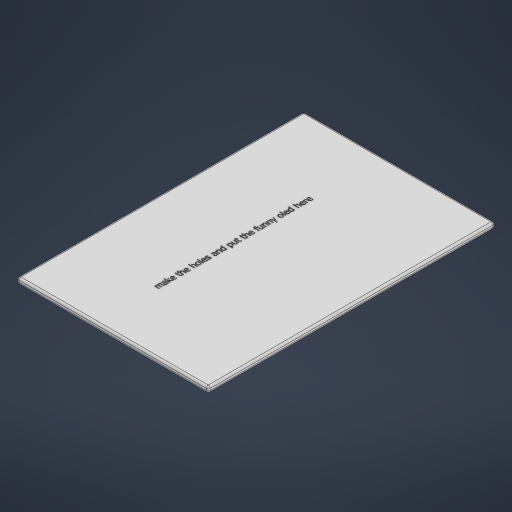
# Autodesk Inventor part: ecu-box-lid
Saved by Autodesk Inventor 2024.2 (Build 282272000, 272)
## iProperties
Created: 2025-06-20
Part Number: ecu-box-lid
Material: Generic
Document SubType Name: Modeling
Designer: Moe
Density: 1 g/cm^3
Appearance: Default
Author: Moe
Autodesk Inventor part; units mm, degrees
(part 1 of 2)
ref_plane "YZ Plane" through (0, 0, 0) normal (1, 0, 0) x (0, 1, 0)
ref_plane "XZ Plane" through (0, 0, 0) normal (0, 1, 0) x (-1, 0, 0)
ref_plane "XY Plane" through (0, 0, 0) normal (0, 0, 1) x (1, 0, 0)
sketch "Sketch1" plane through (0, 0, 0) normal (0, 1, 0) x (-1, 0, 0)
  line L0 (0, 0) -> (100, 0)
  line L1 (100, 0) -> (100, -150)
  line L2 (100, -150) -> (0, -150)
  line L3 (0, -150) -> (0, 0)
  dimension "d0" = 100
  dimension "d1" = 150
  constraints: 8 end point, 2 parallel, 1 horizontal, 1 perpendicular
  measures "d0" distance of L1.end L2.end
  measures "d1" distance of L0.end L1.end
extrude "Extrusion1" add sketch "Sketch1" along normal blind 3
sketch "Sketch2" plane through (0, 0, 0) normal (0, -1, 0) x (1, 0, 0)
  line L0 (0, -150) -> (-100, -150) projected
  line L1 (0, 0) -> (0, -150) projected
  line L2 (-100, 0) -> (0, 0) projected
  line L3 (-100, -150) -> (-100, 0) projected
  line L4 (-5.25, -3.25) -> (-94.75, -3.25)
  line L5 (-96.75, -5.25) -> (-96.75, -144.75)
  line L6 (-94.75, -146.75) -> (-5.25, -146.75)
  line L7 (-3.25, -144.75) -> (-3.25, -5.25)
  arc A0 (-3.25, -5.25) -> (-5.25, -3.25) centre (-5.25, -5.25) ccw
  arc A1 (-94.75, -3.25) -> (-96.75, -5.25) centre (-94.75, -5.25) ccw
  arc A2 (-96.75, -144.75) -> (-94.75, -146.75) centre (-94.75, -144.75) ccw
  arc A3 (-5.25, -146.75) -> (-3.25, -144.75) centre (-5.25, -144.75) ccw
  line L8 (-8.25, -6.25) -> (-91.75, -6.25)
  line L9 (-93.75, -8.25) -> (-93.75, -141.75)
  line L10 (-91.75, -143.75) -> (-8.25, -143.75)
  line L11 (-6.25, -141.75) -> (-6.25, -8.25)
  arc A4 (-6.25, -8.25) -> (-8.25, -6.25) centre (-8.25, -8.25) ccw
  arc A5 (-8.25, -143.75) -> (-6.25, -141.75) centre (-8.25, -141.75) ccw
  arc A6 (-93.75, -141.75) -> (-91.75, -143.75) centre (-91.75, -141.75) ccw
  arc A7 (-91.75, -6.25) -> (-93.75, -8.25) centre (-91.75, -8.25) ccw
  point P0 (-3.25, -3.25)
  point P1 (-96.75, -146.75)
  point P2 (-96.75, -3.25)
  point P3 (-3.25, -146.75)
  point P4 (-50, -143.75)
  dimension "d4" = 3.25
  dimension "d5" = 3.25
  dimension "d6" = 3.25
  dimension "d7" = 3.25
  dimension "d10" = 2
  dimension "d12" = 3
  dimension "d13" = 3
  dimension "d14" = 3
  dimension "d15" = 3
  dimension "d16" = 2
  constraints: 16 end point, 16 point on circle, 16 tangent, 8 centre point, 8 point on line, 6 equal radius, 4 parallel, 2 horizontal, 2 perpendicular, 1 midpoint
  measures "d4" distance between parallel lines of L1 L7
  measures "d5" distance between parallel lines of L3 L5
  measures "d6" distance between parallel lines of L2 L4
  measures "d7" distance between parallel lines of L0 L6
  measures "d10" radius of A0
  measures "d12" distance between parallel lines of L7 L11
  measures "d13" distance between parallel lines of L4 L8
  measures "d14" distance between parallel lines of L5 L9
  measures "d15" distance from line of L6 point (-50, -143.75)
  measures "d16" radius of A4
extrude "Extrusion2" add sketch "Sketch2" along normal blind 3 contours A0 L7 A3 L6 A2 L5 A1 L4
fillet "Fillet1" radius 1 20 edges at (-50, 0, 0) (0, 1.5, 0) (0, 0, -75) (0, 3, -75) (-50, 3, 0) (-3.8358, -3, -3.8358) (-50, -3, -3.25) (-96.1642, -3, -3.8358) (-96.75, -3, -75) (-96.1642, -3, -146.1642) (-50, -3, -146.75) (-3.8358, -3, -146.1642) (-3.25, -3, -75) (0, 1.5, -150) (-50, 3, -150) (-50, 0, -150) (-100, 3, -75) (-100, 1.5, -150) (-100, 0, -75) (-100, 1.5, 0)
sketch "Sketch3" plane through (0, 3, 0) normal (0, 1, 0) x (1, 0, 0)
  line L0 (-60.8151, 31.4553) -> (-60.8151, 114.1441) construction
  line L1 (-60.8151, 114.1441) -> (-56.7693, 114.1441) construction
  line L2 (-56.7693, 114.1441) -> (-56.7693, 31.4553) construction
  line L3 (-56.7693, 31.4553) -> (-60.8151, 31.4553) construction
  line L4 (-57.6115, 34.328) -> (-58.9355, 34.328)
  spline S0 degree 2 poles (-58.9355, 34.328) (-59.0935, 34.328) (-59.3628, 34.3033) (-59.4369, 34.2637) knots 0 0 0 1 2 2 2
  spline S1 degree 2 poles (-59.4369, 34.2637) (-59.5184, 34.2242) (-59.5974, 34.0735) (-59.5974, 33.9426) knots 0 0 0 1 2 2 2
  spline S2 degree 2 poles (-59.5974, 33.9426) (-59.5974, 33.8241) (-59.4517, 33.5524) (-59.3134, 33.4091) knots 0 0 0 1 2 2 2
  spline S3 degree 2 poles (-59.3134, 33.4091) (-59.2788, 33.4116) (-59.1825, 33.4165) (-59.1182, 33.4165) knots 0 0 0 1 2 2 2
  line L5 (-59.1182, 33.4165) -> (-57.6115, 33.4165)
  line L6 (-57.6115, 33.4165) -> (-57.6115, 33.0312)
  line L7 (-57.6115, 33.0312) -> (-58.9355, 33.0312)
  spline S4 degree 2 poles (-58.9355, 33.0312) (-59.0935, 33.0312) (-59.3628, 33.0065) (-59.4369, 32.967) knots 0 0 0 1 2 2 2
  spline S5 degree 2 poles (-59.4369, 32.967) (-59.5184, 32.9275) (-59.5974, 32.7768) (-59.5974, 32.6459) knots 0 0 0 1 2 2 2
  spline S6 degree 2 poles (-59.5974, 32.6459) (-59.5974, 32.5224) (-59.4418, 32.2482) (-59.3208, 32.1198) knots 0 0 0 1 2 2 2
  line L8 (-59.3208, 32.1198) -> (-57.6115, 32.1198)
  line L9 (-57.6115, 32.1198) -> (-57.6115, 31.7344)
  line L10 (-57.6115, 31.7344) -> (-59.8988, 31.7344)
  line L11 (-59.8988, 31.7344) -> (-59.8988, 32.1198)
  line L12 (-59.8988, 32.1198) -> (-59.6468, 32.1198)
  spline S7 degree 2 poles (-59.6468, 32.1198) (-59.7975, 32.2704) (-59.963, 32.5668) (-59.963, 32.7447) knots 0 0 0 1 2 2 2
  spline S8 degree 2 poles (-59.963, 32.7447) (-59.963, 32.9472) (-59.7777, 33.2609) (-59.5678, 33.3424) knots 0 0 0 1 2 2 2
  spline S9 degree 2 poles (-59.5678, 33.3424) (-59.7629, 33.5178) (-59.963, 33.8488) (-59.963, 34.0414) knots 0 0 0 1 2 2 2
  spline S10 degree 2 poles (-59.963, 34.0414) (-59.963, 34.1896) (-59.8716, 34.4317) (-59.7679, 34.5206) knots 0 0 0 1 2 2 2
  spline S11 degree 2 poles (-59.7679, 34.5206) (-59.6641, 34.612) (-59.3529, 34.7133) (-59.1182, 34.7133) knots 0 0 0 1 2 2 2
  line L13 (-59.1182, 34.7133) -> (-57.6115, 34.7133)
  line L14 (-57.6115, 34.7133) -> (-57.6115, 34.328)
  spline S12 degree 2 poles (-57.8536, 36.5287) (-57.819, 36.4818) (-57.6955, 36.3237) (-57.6585, 36.2496) knots 0 0 0 1 2 2 2
  spline S13 degree 2 poles (-57.6585, 36.2496) (-57.6041, 36.1484) (-57.5473, 35.9582) (-57.5473, 35.7853) knots 0 0 0 1 2 2 2
  spline S14 degree 2 poles (-57.5473, 35.7853) (-57.5473, 35.6445) (-57.6535, 35.3901) (-57.7498, 35.2937) knots 0 0 0 1 2 2 2
  spline S15 degree 2 poles (-57.7498, 35.2937) (-57.8437, 35.2023) (-58.1204, 35.0912) (-58.2735, 35.0912) knots 0 0 0 1 2 2 2
  spline S16 degree 2 poles (-58.2735, 35.0912) (-58.5106, 35.0912) (-58.8465, 35.2913) (-58.9429, 35.5086) knots 0 0 0 1 2 2 2
  spline S17 degree 2 poles (-58.9429, 35.5086) (-59.0318, 35.7013) (-59.0985, 36.2249) (-59.1158, 36.5287) knots 0 0 0 1 2 2 2
  line L15 (-59.1158, 36.5287) -> (-59.1899, 36.5287)
  spline S18 degree 2 poles (-59.1899, 36.5287) (-59.3233, 36.5287) (-59.4887, 36.4472) (-59.5357, 36.3731) knots 0 0 0 1 2 2 2
  spline S19 degree 2 poles (-59.5357, 36.3731) (-59.5826, 36.299) (-59.6122, 36.0866) (-59.6122, 35.973) knots 0 0 0 1 2 2 2
  spline S20 degree 2 poles (-59.6122, 35.973) (-59.6122, 35.8396) (-59.5332, 35.479) (-59.4566, 35.2987) knots 0 0 0 1 2 2 2
  line L16 (-59.4566, 35.2987) -> (-59.4566, 35.2764)
  line L17 (-59.4566, 35.2764) -> (-59.8494, 35.2764)
  spline S21 degree 2 poles (-59.8494, 35.2764) (-59.879, 35.3827) (-59.9531, 35.7803) (-59.9531, 35.9755) knots 0 0 0 1 2 2 2
  spline S22 degree 2 poles (-59.9531, 35.9755) (-59.9531, 36.2126) (-59.879, 36.5361) (-59.7827, 36.6646) knots 0 0 0 1 2 2 2
  spline S23 degree 2 poles (-59.7827, 36.6646) (-59.6888, 36.7906) (-59.3899, 36.9141) (-59.175, 36.9141) knots 0 0 0 1 2 2 2
  line L18 (-59.175, 36.9141) -> (-57.6115, 36.9141)
  line L19 (-57.6115, 36.9141) -> (-57.6115, 36.5287)
  line L20 (-57.6115, 36.5287) -> (-57.8536, 36.5287)
  line L21 (-58.1747, 36.5287) -> (-58.8095, 36.5287)
  spline S24 degree 2 poles (-58.8095, 36.5287) (-58.7971, 36.3904) (-58.7551, 35.973) (-58.7156, 35.8421) knots 0 0 0 1 2 2 2
  spline S25 degree 2 poles (-58.7156, 35.8421) (-58.6687, 35.6889) (-58.4736, 35.4889) (-58.3007, 35.4889) knots 0 0 0 1 2 2 2
  spline S26 degree 2 poles (-58.3007, 35.4889) (-58.1031, 35.4889) (-57.903, 35.7112) (-57.903, 35.9236) knots 0 0 0 1 2 2 2
  spline S27 degree 2 poles (-57.903, 35.9236) (-57.903, 36.1039) (-58.0586, 36.4003) (-58.1747, 36.5287) knots 0 0 0 1 2 2 2
  line L22 (-57.6115, 39.3495) -> (-57.6115, 38.8431)
  line L23 (-57.6115, 38.8431) -> (-58.7156, 37.9935)
  line L24 (-58.7156, 37.9935) -> (-58.5674, 37.8403)
  line L25 (-58.5674, 37.8403) -> (-57.6115, 37.8403)
  line L26 (-57.6115, 37.8403) -> (-57.6115, 37.455)
  line L27 (-57.6115, 37.455) -> (-60.7954, 37.455)
  line L28 (-60.7954, 37.455) -> (-60.7954, 37.8403)
  line L29 (-60.7954, 37.8403) -> (-58.933, 37.8403)
  line L30 (-58.933, 37.8403) -> (-59.8988, 38.7443)
  line L31 (-59.8988, 38.7443) -> (-59.8988, 39.2235)
  line L32 (-59.8988, 39.2235) -> (-58.9429, 38.2849)
  line L33 (-58.9429, 38.2849) -> (-57.6115, 39.3495)
  spline S28 degree 2 poles (-57.5597, 40.5351) (-57.5597, 39.9868) (-58.1747, 39.3841) (-58.7428, 39.3841) knots 0 0 0 1 2 2 2
  spline S29 degree 2 poles (-58.7428, 39.3841) (-59.301, 39.3841) (-59.963, 39.9695) (-59.963, 40.4412) knots 0 0 0 1 2 2 2
  spline S30 degree 2 poles (-59.963, 40.4412) (-59.963, 40.6537) (-59.8395, 40.9822) (-59.7086, 41.1032) knots 0 0 0 1 2 2 2
  spline S31 degree 2 poles (-59.7086, 41.1032) (-59.5777, 41.2267) (-59.1997, 41.3576) (-58.9256, 41.3576) knots 0 0 0 1 2 2 2
  line L34 (-58.9256, 41.3576) -> (-58.7156, 41.3576)
  line L35 (-58.7156, 41.3576) -> (-58.7156, 39.7743)
  spline S32 degree 2 poles (-58.7156, 39.7743) (-58.318, 39.7743) (-57.8956, 40.1745) (-57.8956, 40.5302) knots 0 0 0 1 2 2 2
  spline S33 degree 2 poles (-57.8956, 40.5302) (-57.8956, 40.6561) (-57.9524, 40.9007) (-57.9969, 40.9995) knots 0 0 0 1 2 2 2
  spline S34 degree 2 poles (-57.9969, 40.9995) (-58.0463, 41.1032) (-58.1327, 41.2465) (-58.1722, 41.2934) knots 0 0 0 1 2 2 2
  line L36 (-58.1722, 41.2934) -> (-58.1722, 41.3156)
  line L37 (-58.1722, 41.3156) -> (-57.7523, 41.3156)
  spline S35 degree 2 poles (-57.7523, 41.3156) (-57.7251, 41.2489) (-57.6461, 41.0464) (-57.6239, 40.9674) knots 0 0 0 1 2 2 2
  spline S36 degree 2 poles (-57.6239, 40.9674) (-57.5918, 40.8562) (-57.5597, 40.6734) (-57.5597, 40.5351) knots 0 0 0 1 2 2 2
  spline S37 degree 2 poles (-59.0096, 40.9822) (-59.1652, 40.9772) (-59.3924, 40.913) (-59.469, 40.8513) knots 0 0 0 1 2 2 2
  spline S38 degree 2 poles (-59.469, 40.8513) (-59.5554, 40.7846) (-59.6468, 40.5746) (-59.6468, 40.419) knots 0 0 0 1 2 2 2
  spline S39 degree 2 poles (-59.6468, 40.419) (-59.6468, 40.2659) (-59.5554, 40.051) (-59.4665, 39.9621) knots 0 0 0 1 2 2 2
  spline S40 degree 2 poles (-59.4665, 39.9621) (-59.3751, 39.8756) (-59.1553, 39.7867) (-59.0096, 39.7743) knots 0 0 0 1 2 2 2
  line L38 (-59.0096, 39.7743) -> (-59.0096, 40.9822)
  spline S41 degree 2 poles (-57.5671, 43.7486) (-57.5671, 43.4349) (-57.9252, 43.0817) (-58.313, 43.0817) knots 0 0 0 1 2 2 2
  line L39 (-58.313, 43.0817) -> (-59.5801, 43.0817)
  line L40 (-59.5801, 43.0817) -> (-59.5801, 42.8223)
  line L41 (-59.5801, 42.8223) -> (-59.8988, 42.8223)
  line L42 (-59.8988, 42.8223) -> (-59.8988, 43.0817)
  line L43 (-59.8988, 43.0817) -> (-60.5558, 43.0817)
  line L44 (-60.5558, 43.0817) -> (-60.5558, 43.467)
  line L45 (-60.5558, 43.467) -> (-59.8988, 43.467)
  line L46 (-59.8988, 43.467) -> (-59.8988, 44.1759)
  line L47 (-59.8988, 44.1759) -> (-59.5801, 44.1759)
  line L48 (-59.5801, 44.1759) -> (-59.5801, 43.467)
  line L49 (-59.5801, 43.467) -> (-58.4909, 43.467)
  spline S42 degree 2 poles (-58.4909, 43.467) (-58.318, 43.467) (-58.1278, 43.4794) (-58.0463, 43.5214) knots 0 0 0 1 2 2 2
  spline S43 degree 2 poles (-58.0463, 43.5214) (-57.9746, 43.5559) (-57.903, 43.7115) (-57.903, 43.8449) knots 0 0 0 1 2 2 2
  spline S44 degree 2 poles (-57.903, 43.8449) (-57.903, 43.9388) (-57.9598, 44.1142) (-57.9771, 44.1537) knots 0 0 0 1 2 2 2
  line L50 (-57.9771, 44.1537) -> (-57.9771, 44.1759)
  line L51 (-57.9771, 44.1759) -> (-57.6313, 44.1759)
  spline S45 degree 2 poles (-57.6313, 44.1759) (-57.6016, 44.0672) (-57.5671, 43.8449) (-57.5671, 43.7486) knots 0 0 0 1 2 2 2
  line L52 (-57.6115, 46.2557) -> (-57.6115, 45.8703)
  line L53 (-57.6115, 45.8703) -> (-58.9157, 45.8703)
  spline S46 degree 2 poles (-58.9157, 45.8703) (-59.0738, 45.8703) (-59.3455, 45.8407) (-59.427, 45.7962) knots 0 0 0 1 2 2 2
  spline S47 degree 2 poles (-59.427, 45.7962) (-59.5134, 45.7493) (-59.5974, 45.5813) (-59.5974, 45.4381) knots 0 0 0 1 2 2 2
  spline S48 degree 2 poles (-59.5974, 45.4381) (-59.5974, 45.2948) (-59.4443, 44.991) (-59.3208, 44.8453) knots 0 0 0 1 2 2 2
  line L54 (-59.3208, 44.8453) -> (-57.6115, 44.8453)
  line L55 (-57.6115, 44.8453) -> (-57.6115, 44.46)
  line L56 (-57.6115, 44.46) -> (-60.7954, 44.46)
  line L57 (-60.7954, 44.46) -> (-60.7954, 44.8453)
  line L58 (-60.7954, 44.8453) -> (-59.6444, 44.8453)
  spline S49 degree 2 poles (-59.6444, 44.8453) (-59.8, 45.0182) (-59.963, 45.3516) (-59.963, 45.5394) knots 0 0 0 1 2 2 2
  spline S50 degree 2 poles (-59.963, 45.5394) (-59.963, 45.8753) (-59.5184, 46.2557) (-59.096, 46.2557) knots 0 0 0 1 2 2 2
  line L59 (-59.096, 46.2557) -> (-57.6115, 46.2557)
  spline S51 degree 2 poles (-57.5597, 47.7895) (-57.5597, 47.2412) (-58.1747, 46.6385) (-58.7428, 46.6385) knots 0 0 0 1 2 2 2
  spline S52 degree 2 poles (-58.7428, 46.6385) (-59.301, 46.6385) (-59.963, 47.2239) (-59.963, 47.6957) knots 0 0 0 1 2 2 2
  spline S53 degree 2 poles (-59.963, 47.6957) (-59.963, 47.9081) (-59.8395, 48.2366) (-59.7086, 48.3576) knots 0 0 0 1 2 2 2
  spline S54 degree 2 poles (-59.7086, 48.3576) (-59.5777, 48.4811) (-59.1997, 48.6121) (-58.9256, 48.6121) knots 0 0 0 1 2 2 2
  line L60 (-58.9256, 48.6121) -> (-58.7156, 48.6121)
  line L61 (-58.7156, 48.6121) -> (-58.7156, 47.0288)
  spline S55 degree 2 poles (-58.7156, 47.0288) (-58.318, 47.0288) (-57.8956, 47.4289) (-57.8956, 47.7846) knots 0 0 0 1 2 2 2
  spline S56 degree 2 poles (-57.8956, 47.7846) (-57.8956, 47.9106) (-57.9524, 48.1551) (-57.9969, 48.2539) knots 0 0 0 1 2 2 2
  spline S57 degree 2 poles (-57.9969, 48.2539) (-58.0463, 48.3576) (-58.1327, 48.5009) (-58.1722, 48.5478) knots 0 0 0 1 2 2 2
  line L62 (-58.1722, 48.5478) -> (-58.1722, 48.5701)
  line L63 (-58.1722, 48.5701) -> (-57.7523, 48.5701)
  spline S58 degree 2 poles (-57.7523, 48.5701) (-57.7251, 48.5034) (-57.6461, 48.3008) (-57.6239, 48.2218) knots 0 0 0 1 2 2 2
  spline S59 degree 2 poles (-57.6239, 48.2218) (-57.5918, 48.1106) (-57.5597, 47.9279) (-57.5597, 47.7895) knots 0 0 0 1 2 2 2
  spline S60 degree 2 poles (-59.0096, 48.2366) (-59.1652, 48.2317) (-59.3924, 48.1675) (-59.469, 48.1057) knots 0 0 0 1 2 2 2
  spline S61 degree 2 poles (-59.469, 48.1057) (-59.5554, 48.039) (-59.6468, 47.8291) (-59.6468, 47.6735) knots 0 0 0 1 2 2 2
  spline S62 degree 2 poles (-59.6468, 47.6735) (-59.6468, 47.5203) (-59.5554, 47.3054) (-59.4665, 47.2165) knots 0 0 0 1 2 2 2
  spline S63 degree 2 poles (-59.4665, 47.2165) (-59.3751, 47.13) (-59.1553, 47.0411) (-59.0096, 47.0288) knots 0 0 0 1 2 2 2
  line L64 (-59.0096, 47.0288) -> (-59.0096, 48.2366)
  line L65 (-57.6115, 52.1071) -> (-57.6115, 51.7218)
  line L66 (-57.6115, 51.7218) -> (-58.9157, 51.7218)
  spline S64 degree 2 poles (-58.9157, 51.7218) (-59.0738, 51.7218) (-59.3455, 51.6922) (-59.427, 51.6477) knots 0 0 0 1 2 2 2
  spline S65 degree 2 poles (-59.427, 51.6477) (-59.5134, 51.6008) (-59.5974, 51.4328) (-59.5974, 51.2896) knots 0 0 0 1 2 2 2
  spline S66 degree 2 poles (-59.5974, 51.2896) (-59.5974, 51.1463) (-59.4443, 50.8425) (-59.3208, 50.6968) knots 0 0 0 1 2 2 2
  line L67 (-59.3208, 50.6968) -> (-57.6115, 50.6968)
  line L68 (-57.6115, 50.6968) -> (-57.6115, 50.3114)
  line L69 (-57.6115, 50.3114) -> (-60.7954, 50.3114)
  line L70 (-60.7954, 50.3114) -> (-60.7954, 50.6968)
  line L71 (-60.7954, 50.6968) -> (-59.6444, 50.6968)
  spline S67 degree 2 poles (-59.6444, 50.6968) (-59.8, 50.8697) (-59.963, 51.2031) (-59.963, 51.3908) knots 0 0 0 1 2 2 2
  spline S68 degree 2 poles (-59.963, 51.3908) (-59.963, 51.7267) (-59.5184, 52.1071) (-59.096, 52.1071) knots 0 0 0 1 2 2 2
  line L72 (-59.096, 52.1071) -> (-57.6115, 52.1071)
  spline S69 degree 2 poles (-58.7551, 54.5277) (-58.1772, 54.5277) (-57.5473, 53.972) (-57.5473, 53.5076) knots 0 0 0 1 2 2 2
  spline S70 degree 2 poles (-57.5473, 53.5076) (-57.5473, 53.0309) (-58.1969, 52.485) (-58.7551, 52.485) knots 0 0 0 1 2 2 2
  spline S71 degree 2 poles (-58.7551, 52.485) (-59.3282, 52.485) (-59.963, 53.0482) (-59.963, 53.5076) knots 0 0 0 1 2 2 2
  spline S72 degree 2 poles (-59.963, 53.5076) (-59.963, 53.972) (-59.3307, 54.5277) (-58.7551, 54.5277) knots 0 0 0 1 2 2 2
  spline S73 degree 2 poles (-58.7551, 54.1301) (-59.1997, 54.1301) (-59.632, 53.8065) (-59.632, 53.5076) knots 0 0 0 1 2 2 2
  spline S74 degree 2 poles (-59.632, 53.5076) (-59.632, 53.2088) (-59.1997, 52.8827) (-58.7551, 52.8827) knots 0 0 0 1 2 2 2
  spline S75 degree 2 poles (-58.7551, 52.8827) (-58.3229, 52.8827) (-57.8783, 53.2088) (-57.8783, 53.5076) knots 0 0 0 1 2 2 2
  spline S76 degree 2 poles (-57.8783, 53.5076) (-57.8783, 53.804) (-58.3155, 54.1301) (-58.7551, 54.1301) knots 0 0 0 1 2 2 2
  line L73 (-57.6115, 55.3157) -> (-57.6115, 54.9304)
  line L74 (-57.6115, 54.9304) -> (-60.7954, 54.9304)
  line L75 (-60.7954, 54.9304) -> (-60.7954, 55.3157)
  line L76 (-60.7954, 55.3157) -> (-57.6115, 55.3157)
  spline S77 degree 2 poles (-57.5597, 56.8743) (-57.5597, 56.3259) (-58.1747, 55.7232) (-58.7428, 55.7232) knots 0 0 0 1 2 2 2
  spline S78 degree 2 poles (-58.7428, 55.7232) (-59.301, 55.7232) (-59.963, 56.3086) (-59.963, 56.7804) knots 0 0 0 1 2 2 2
  spline S79 degree 2 poles (-59.963, 56.7804) (-59.963, 56.9928) (-59.8395, 57.3213) (-59.7086, 57.4424) knots 0 0 0 1 2 2 2
  spline S80 degree 2 poles (-59.7086, 57.4424) (-59.5777, 57.5659) (-59.1997, 57.6968) (-58.9256, 57.6968) knots 0 0 0 1 2 2 2
  line L77 (-58.9256, 57.6968) -> (-58.7156, 57.6968)
  line L78 (-58.7156, 57.6968) -> (-58.7156, 56.1135)
  spline S81 degree 2 poles (-58.7156, 56.1135) (-58.318, 56.1135) (-57.8956, 56.5136) (-57.8956, 56.8693) knots 0 0 0 1 2 2 2
  spline S82 degree 2 poles (-57.8956, 56.8693) (-57.8956, 56.9953) (-57.9524, 57.2398) (-57.9969, 57.3386) knots 0 0 0 1 2 2 2
  spline S83 degree 2 poles (-57.9969, 57.3386) (-58.0463, 57.4424) (-58.1327, 57.5856) (-58.1722, 57.6326) knots 0 0 0 1 2 2 2
  line L79 (-58.1722, 57.6326) -> (-58.1722, 57.6548)
  line L80 (-58.1722, 57.6548) -> (-57.7523, 57.6548)
  spline S84 degree 2 poles (-57.7523, 57.6548) (-57.7251, 57.5881) (-57.6461, 57.3856) (-57.6239, 57.3065) knots 0 0 0 1 2 2 2
  spline S85 degree 2 poles (-57.6239, 57.3065) (-57.5918, 57.1954) (-57.5597, 57.0126) (-57.5597, 56.8743) knots 0 0 0 1 2 2 2
  spline S86 degree 2 poles (-59.0096, 57.3213) (-59.1652, 57.3164) (-59.3924, 57.2522) (-59.469, 57.1904) knots 0 0 0 1 2 2 2
  spline S87 degree 2 poles (-59.469, 57.1904) (-59.5554, 57.1237) (-59.6468, 56.9138) (-59.6468, 56.7582) knots 0 0 0 1 2 2 2
  spline S88 degree 2 poles (-59.6468, 56.7582) (-59.6468, 56.605) (-59.5554, 56.3901) (-59.4665, 56.3012) knots 0 0 0 1 2 2 2
  spline S89 degree 2 poles (-59.4665, 56.3012) (-59.3751, 56.2148) (-59.1553, 56.1258) (-59.0096, 56.1135) knots 0 0 0 1 2 2 2
  line L81 (-59.0096, 56.1135) -> (-59.0096, 57.3213)
  spline S90 degree 2 poles (-57.5572, 58.7045) (-57.5572, 58.4748) (-57.6807, 58.0772) (-57.7498, 57.9463) knots 0 0 0 1 2 2 2
  line L82 (-57.7498, 57.9463) -> (-58.1821, 57.9463)
  line L83 (-58.1821, 57.9463) -> (-58.1821, 57.966)
  spline S91 degree 2 poles (-58.1821, 57.966) (-58.1426, 58.0154) (-58.0487, 58.1488) (-57.9969, 58.2599) knots 0 0 0 1 2 2 2
  spline S92 degree 2 poles (-57.9969, 58.2599) (-57.9499, 58.3563) (-57.8808, 58.5934) (-57.8808, 58.7194) knots 0 0 0 1 2 2 2
  spline S93 degree 2 poles (-57.8808, 58.7194) (-57.8808, 58.8108) (-57.9228, 59.0207) (-57.9573, 59.0701) knots 0 0 0 1 2 2 2
  spline S94 degree 2 poles (-57.9573, 59.0701) (-58.0043, 59.1417) (-58.1105, 59.206) (-58.2192, 59.206) knots 0 0 0 1 2 2 2
  spline S95 degree 2 poles (-58.2192, 59.206) (-58.355, 59.206) (-58.4958, 59.0578) (-58.5427, 58.8676) knots 0 0 0 1 2 2 2
  spline S96 degree 2 poles (-58.5427, 58.8676) (-58.56, 58.7935) (-58.6094, 58.5563) (-58.6366, 58.4551) knots 0 0 0 1 2 2 2
  spline S97 degree 2 poles (-58.6366, 58.4551) (-58.7132, 58.1933) (-59.0293, 57.9561) (-59.2541, 57.9561) knots 0 0 0 1 2 2 2
  spline S98 degree 2 poles (-59.2541, 57.9561) (-59.5653, 57.9561) (-59.9531, 58.423) (-59.9531, 58.8083) knots 0 0 0 1 2 2 2
  spline S99 degree 2 poles (-59.9531, 58.8083) (-59.9531, 58.9985) (-59.8592, 59.3838) (-59.7876, 59.5147) knots 0 0 0 1 2 2 2
  line L84 (-59.7876, 59.5147) -> (-59.3751, 59.5147)
  line L85 (-59.3751, 59.5147) -> (-59.3751, 59.495)
  spline S100 degree 2 poles (-59.3751, 59.495) (-59.4937, 59.3467) (-59.6295, 58.9861) (-59.6295, 58.8009) knots 0 0 0 1 2 2 2
  spline S101 degree 2 poles (-59.6295, 58.8009) (-59.6295, 58.6107) (-59.469, 58.3489) (-59.3084, 58.3489) knots 0 0 0 1 2 2 2
  spline S102 degree 2 poles (-59.3084, 58.3489) (-59.1627, 58.3489) (-59.0219, 58.5045) (-58.9774, 58.6774) knots 0 0 0 1 2 2 2
  spline S103 degree 2 poles (-58.9774, 58.6774) (-58.9552, 58.7614) (-58.9108, 58.9738) (-58.8836, 59.0899) knots 0 0 0 1 2 2 2
  spline S104 degree 2 poles (-58.8836, 59.0899) (-58.8194, 59.3418) (-58.5254, 59.5987) (-58.271, 59.5987) knots 0 0 0 1 2 2 2
  spline S105 degree 2 poles (-58.271, 59.5987) (-58.1228, 59.5987) (-57.861, 59.4826) (-57.7647, 59.369) knots 0 0 0 1 2 2 2
  spline S106 degree 2 poles (-57.7647, 59.369) (-57.6634, 59.2479) (-57.5572, 58.9392) (-57.5572, 58.7045) knots 0 0 0 1 2 2 2
  spline S107 degree 2 poles (-57.8536, 62.5405) (-57.819, 62.4936) (-57.6955, 62.3355) (-57.6585, 62.2614) knots 0 0 0 1 2 2 2
  spline S108 degree 2 poles (-57.6585, 62.2614) (-57.6041, 62.1601) (-57.5473, 61.9699) (-57.5473, 61.797) knots 0 0 0 1 2 2 2
  spline S109 degree 2 poles (-57.5473, 61.797) (-57.5473, 61.6562) (-57.6535, 61.4018) (-57.7498, 61.3055) knots 0 0 0 1 2 2 2
  spline S110 degree 2 poles (-57.7498, 61.3055) (-57.8437, 61.2141) (-58.1204, 61.1029) (-58.2735, 61.1029) knots 0 0 0 1 2 2 2
  spline S111 degree 2 poles (-58.2735, 61.1029) (-58.5106, 61.1029) (-58.8465, 61.303) (-58.9429, 61.5204) knots 0 0 0 1 2 2 2
  spline S112 degree 2 poles (-58.9429, 61.5204) (-59.0318, 61.713) (-59.0985, 62.2367) (-59.1158, 62.5405) knots 0 0 0 1 2 2 2
  line L86 (-59.1158, 62.5405) -> (-59.1899, 62.5405)
  spline S113 degree 2 poles (-59.1899, 62.5405) (-59.3233, 62.5405) (-59.4887, 62.459) (-59.5357, 62.3849) knots 0 0 0 1 2 2 2
  spline S114 degree 2 poles (-59.5357, 62.3849) (-59.5826, 62.3108) (-59.6122, 62.0983) (-59.6122, 61.9847) knots 0 0 0 1 2 2 2
  spline S115 degree 2 poles (-59.6122, 61.9847) (-59.6122, 61.8513) (-59.5332, 61.4907) (-59.4566, 61.3104) knots 0 0 0 1 2 2 2
  line L87 (-59.4566, 61.3104) -> (-59.4566, 61.2882)
  line L88 (-59.4566, 61.2882) -> (-59.8494, 61.2882)
  spline S116 degree 2 poles (-59.8494, 61.2882) (-59.879, 61.3944) (-59.9531, 61.7921) (-59.9531, 61.9872) knots 0 0 0 1 2 2 2
  spline S117 degree 2 poles (-59.9531, 61.9872) (-59.9531, 62.2243) (-59.879, 62.5479) (-59.7827, 62.6763) knots 0 0 0 1 2 2 2
  spline S118 degree 2 poles (-59.7827, 62.6763) (-59.6888, 62.8023) (-59.3899, 62.9258) (-59.175, 62.9258) knots 0 0 0 1 2 2 2
  line L89 (-59.175, 62.9258) -> (-57.6115, 62.9258)
  line L90 (-57.6115, 62.9258) -> (-57.6115, 62.5405)
  line L91 (-57.6115, 62.5405) -> (-57.8536, 62.5405)
  line L92 (-58.1747, 62.5405) -> (-58.8095, 62.5405)
  spline S119 degree 2 poles (-58.8095, 62.5405) (-58.7971, 62.4022) (-58.7551, 61.9847) (-58.7156, 61.8538) knots 0 0 0 1 2 2 2
  spline S120 degree 2 poles (-58.7156, 61.8538) (-58.6687, 61.7007) (-58.4736, 61.5006) (-58.3007, 61.5006) knots 0 0 0 1 2 2 2
  spline S121 degree 2 poles (-58.3007, 61.5006) (-58.1031, 61.5006) (-57.903, 61.7229) (-57.903, 61.9353) knots 0 0 0 1 2 2 2
  spline S122 degree 2 poles (-57.903, 61.9353) (-57.903, 62.1156) (-58.0586, 62.412) (-58.1747, 62.5405) knots 0 0 0 1 2 2 2
  line L93 (-57.6115, 65.2624) -> (-57.6115, 64.8771)
  line L94 (-57.6115, 64.8771) -> (-58.9157, 64.8771)
  spline S123 degree 2 poles (-58.9157, 64.8771) (-59.0738, 64.8771) (-59.3455, 64.8475) (-59.427, 64.803) knots 0 0 0 1 2 2 2
  spline S124 degree 2 poles (-59.427, 64.803) (-59.5134, 64.7561) (-59.5974, 64.5881) (-59.5974, 64.4449) knots 0 0 0 1 2 2 2
  spline S125 degree 2 poles (-59.5974, 64.4449) (-59.5974, 64.3016) (-59.4443, 63.9978) (-59.3208, 63.8521) knots 0 0 0 1 2 2 2
  line L95 (-59.3208, 63.8521) -> (-57.6115, 63.8521)
  line L96 (-57.6115, 63.8521) -> (-57.6115, 63.4667)
  line L97 (-57.6115, 63.4667) -> (-59.8988, 63.4667)
  line L98 (-59.8988, 63.4667) -> (-59.8988, 63.8521)
  line L99 (-59.8988, 63.8521) -> (-59.6444, 63.8521)
  spline S126 degree 2 poles (-59.6444, 63.8521) (-59.8, 64.025) (-59.963, 64.3584) (-59.963, 64.5461) knots 0 0 0 1 2 2 2
  spline S127 degree 2 poles (-59.963, 64.5461) (-59.963, 64.8821) (-59.5184, 65.2624) (-59.096, 65.2624) knots 0 0 0 1 2 2 2
  line L100 (-59.096, 65.2624) -> (-57.6115, 65.2624)
  line L101 (-57.6115, 67.562) -> (-57.6115, 67.1767)
  line L102 (-57.6115, 67.1767) -> (-57.8437, 67.1767)
  spline S128 degree 2 poles (-57.8437, 67.1767) (-57.7696, 67.0878) (-57.6708, 66.9569) (-57.6288, 66.8679) knots 0 0 0 1 2 2 2
  spline S129 degree 2 poles (-57.6288, 66.8679) (-57.5893, 66.7864) (-57.5473, 66.6111) (-57.5473, 66.495) knots 0 0 0 1 2 2 2
  spline S130 degree 2 poles (-57.5473, 66.495) (-57.5473, 66.3073) (-57.7029, 65.9911) (-57.8536, 65.8799) knots 0 0 0 1 2 2 2
  spline S131 degree 2 poles (-57.8536, 65.8799) (-58.0043, 65.7688) (-58.4489, 65.6453) (-58.7379, 65.6453) knots 0 0 0 1 2 2 2
  spline S132 degree 2 poles (-58.7379, 65.6453) (-59.0392, 65.6453) (-59.4789, 65.8009) (-59.6444, 65.9368) knots 0 0 0 1 2 2 2
  spline S133 degree 2 poles (-59.6444, 65.9368) (-59.7926, 66.0627) (-59.963, 66.4159) (-59.963, 66.6111) knots 0 0 0 1 2 2 2
  spline S134 degree 2 poles (-59.963, 66.6111) (-59.963, 66.7815) (-59.8864, 67.0359) (-59.8074, 67.1767) knots 0 0 0 1 2 2 2
  line L103 (-59.8074, 67.1767) -> (-60.7954, 67.1767)
  line L104 (-60.7954, 67.1767) -> (-60.7954, 67.562)
  line L105 (-60.7954, 67.562) -> (-57.6115, 67.562)
  line L106 (-58.1673, 67.1767) -> (-59.4887, 67.1767)
  spline S135 degree 2 poles (-59.4887, 67.1767) (-59.5579, 67.0334) (-59.6098, 66.8062) (-59.6098, 66.6753) knots 0 0 0 1 2 2 2
  spline S136 degree 2 poles (-59.6098, 66.6753) (-59.6098, 66.3789) (-59.1652, 66.043) (-58.7453, 66.043) knots 0 0 0 1 2 2 2
  spline S137 degree 2 poles (-58.7453, 66.043) (-58.3402, 66.043) (-57.9129, 66.2998) (-57.9129, 66.5839) knots 0 0 0 1 2 2 2
  spline S138 degree 2 poles (-57.9129, 66.5839) (-57.9129, 66.7346) (-58.0512, 67.0409) (-58.1673, 67.1767) knots 0 0 0 1 2 2 2
  spline S139 degree 2 poles (-58.8169, 71.3461) (-58.2439, 71.3461) (-57.5671, 70.8002) (-57.5671, 70.3828) knots 0 0 0 1 2 2 2
  spline S140 degree 2 poles (-57.5671, 70.3828) (-57.5671, 70.2124) (-57.6461, 69.9505) (-57.7276, 69.8147) knots 0 0 0 1 2 2 2
  line L107 (-57.7276, 69.8147) -> (-56.7693, 69.8147)
  line L108 (-56.7693, 69.8147) -> (-56.7693, 69.4294)
  line L109 (-56.7693, 69.4294) -> (-59.8988, 69.4294)
  line L110 (-59.8988, 69.4294) -> (-59.8988, 69.8147)
  line L111 (-59.8988, 69.8147) -> (-59.6592, 69.8147)
  spline S141 degree 2 poles (-59.6592, 69.8147) (-59.7901, 69.9579) (-59.963, 70.3087) (-59.963, 70.5137) knots 0 0 0 1 2 2 2
  spline S142 degree 2 poles (-59.963, 70.5137) (-59.963, 70.9064) (-59.3405, 71.3461) (-58.8169, 71.3461) knots 0 0 0 1 2 2 2
  spline S143 degree 2 poles (-58.7724, 70.9484) (-59.1652, 70.9484) (-59.5974, 70.6989) (-59.5974, 70.4198) knots 0 0 0 1 2 2 2
  spline S144 degree 2 poles (-59.5974, 70.4198) (-59.5974, 70.2568) (-59.4517, 69.9505) (-59.3381, 69.8147) knots 0 0 0 1 2 2 2
  line L112 (-59.3381, 69.8147) -> (-58.0388, 69.8147)
  spline S145 degree 2 poles (-58.0388, 69.8147) (-57.9672, 69.9653) (-57.9129, 70.1802) (-57.9129, 70.3186) knots 0 0 0 1 2 2 2
  spline S146 degree 2 poles (-57.9129, 70.3186) (-57.9129, 70.6174) (-58.3525, 70.9484) (-58.7724, 70.9484) knots 0 0 0 1 2 2 2
  line L113 (-57.6115, 73.5246) -> (-57.6115, 73.1393)
  line L114 (-57.6115, 73.1393) -> (-57.8635, 73.1393)
  spline S147 degree 2 poles (-57.8635, 73.1393) (-57.7079, 72.9615) (-57.5473, 72.6428) (-57.5473, 72.4452) knots 0 0 0 1 2 2 2
  spline S148 degree 2 poles (-57.5473, 72.4452) (-57.5473, 72.297) (-57.6461, 72.0328) (-57.7523, 71.9364) knots 0 0 0 1 2 2 2
  spline S149 degree 2 poles (-57.7523, 71.9364) (-57.8585, 71.8376) (-58.1821, 71.7289) (-58.4143, 71.7289) knots 0 0 0 1 2 2 2
  line L115 (-58.4143, 71.7289) -> (-59.8988, 71.7289)
  line L116 (-59.8988, 71.7289) -> (-59.8988, 72.1143)
  line L117 (-59.8988, 72.1143) -> (-58.5946, 72.1143)
  spline S150 degree 2 poles (-58.5946, 72.1143) (-58.4118, 72.1143) (-58.1722, 72.1414) (-58.0833, 72.1884) knots 0 0 0 1 2 2 2
  spline S151 degree 2 poles (-58.0833, 72.1884) (-57.9944, 72.2353) (-57.9129, 72.3958) (-57.9129, 72.5465) knots 0 0 0 1 2 2 2
  spline S152 degree 2 poles (-57.9129, 72.5465) (-57.9129, 72.6873) (-58.0734, 73.0059) (-58.1895, 73.1393) knots 0 0 0 1 2 2 2
  line L118 (-58.1895, 73.1393) -> (-59.8988, 73.1393)
  line L119 (-59.8988, 73.1393) -> (-59.8988, 73.5246)
  line L120 (-59.8988, 73.5246) -> (-57.6115, 73.5246)
  spline S153 degree 2 poles (-57.5671, 74.7745) (-57.5671, 74.4608) (-57.9252, 74.1076) (-58.313, 74.1076) knots 0 0 0 1 2 2 2
  line L121 (-58.313, 74.1076) -> (-59.5801, 74.1076)
  line L122 (-59.5801, 74.1076) -> (-59.5801, 73.8482)
  line L123 (-59.5801, 73.8482) -> (-59.8988, 73.8482)
  line L124 (-59.8988, 73.8482) -> (-59.8988, 74.1076)
  line L125 (-59.8988, 74.1076) -> (-60.5558, 74.1076)
  line L126 (-60.5558, 74.1076) -> (-60.5558, 74.4929)
  line L127 (-60.5558, 74.4929) -> (-59.8988, 74.4929)
  line L128 (-59.8988, 74.4929) -> (-59.8988, 75.2018)
  line L129 (-59.8988, 75.2018) -> (-59.5801, 75.2018)
  line L130 (-59.5801, 75.2018) -> (-59.5801, 74.4929)
  line L131 (-59.5801, 74.4929) -> (-58.4909, 74.4929)
  spline S154 degree 2 poles (-58.4909, 74.4929) (-58.318, 74.4929) (-58.1278, 74.5052) (-58.0463, 74.5472) knots 0 0 0 1 2 2 2
  spline S155 degree 2 poles (-58.0463, 74.5472) (-57.9746, 74.5818) (-57.903, 74.7374) (-57.903, 74.8708) knots 0 0 0 1 2 2 2
  spline S156 degree 2 poles (-57.903, 74.8708) (-57.903, 74.9647) (-57.9598, 75.14) (-57.9771, 75.1796) knots 0 0 0 1 2 2 2
  line L132 (-57.9771, 75.1796) -> (-57.9771, 75.2018)
  line L133 (-57.9771, 75.2018) -> (-57.6313, 75.2018)
  spline S157 degree 2 poles (-57.6313, 75.2018) (-57.6016, 75.0931) (-57.5671, 74.8708) (-57.5671, 74.7745) knots 0 0 0 1 2 2 2
  spline S158 degree 2 poles (-57.5671, 77.4865) (-57.5671, 77.1729) (-57.9252, 76.8196) (-58.313, 76.8196) knots 0 0 0 1 2 2 2
  line L134 (-58.313, 76.8196) -> (-59.5801, 76.8196)
  line L135 (-59.5801, 76.8196) -> (-59.5801, 76.5603)
  line L136 (-59.5801, 76.5603) -> (-59.8988, 76.5603)
  line L137 (-59.8988, 76.5603) -> (-59.8988, 76.8196)
  line L138 (-59.8988, 76.8196) -> (-60.5558, 76.8196)
  line L139 (-60.5558, 76.8196) -> (-60.5558, 77.205)
  line L140 (-60.5558, 77.205) -> (-59.8988, 77.205)
  line L141 (-59.8988, 77.205) -> (-59.8988, 77.9139)
  line L142 (-59.8988, 77.9139) -> (-59.5801, 77.9139)
  line L143 (-59.5801, 77.9139) -> (-59.5801, 77.205)
  line L144 (-59.5801, 77.205) -> (-58.4909, 77.205)
  spline S159 degree 2 poles (-58.4909, 77.205) (-58.318, 77.205) (-58.1278, 77.2173) (-58.0463, 77.2593) knots 0 0 0 1 2 2 2
  spline S160 degree 2 poles (-58.0463, 77.2593) (-57.9746, 77.2939) (-57.903, 77.4495) (-57.903, 77.5829) knots 0 0 0 1 2 2 2
  spline S161 degree 2 poles (-57.903, 77.5829) (-57.903, 77.6767) (-57.9598, 77.8521) (-57.9771, 77.8916) knots 0 0 0 1 2 2 2
  line L145 (-57.9771, 77.8916) -> (-57.9771, 77.9139)
  line L146 (-57.9771, 77.9139) -> (-57.6313, 77.9139)
  spline S162 degree 2 poles (-57.6313, 77.9139) (-57.6016, 77.8052) (-57.5671, 77.5829) (-57.5671, 77.4865) knots 0 0 0 1 2 2 2
  line L147 (-57.6115, 79.9936) -> (-57.6115, 79.6083)
  line L148 (-57.6115, 79.6083) -> (-58.9157, 79.6083)
  spline S163 degree 2 poles (-58.9157, 79.6083) (-59.0738, 79.6083) (-59.3455, 79.5787) (-59.427, 79.5342) knots 0 0 0 1 2 2 2
  spline S164 degree 2 poles (-59.427, 79.5342) (-59.5134, 79.4873) (-59.5974, 79.3193) (-59.5974, 79.176) knots 0 0 0 1 2 2 2
  spline S165 degree 2 poles (-59.5974, 79.176) (-59.5974, 79.0328) (-59.4443, 78.729) (-59.3208, 78.5832) knots 0 0 0 1 2 2 2
  line L149 (-59.3208, 78.5832) -> (-57.6115, 78.5832)
  line L150 (-57.6115, 78.5832) -> (-57.6115, 78.1979)
  line L151 (-57.6115, 78.1979) -> (-60.7954, 78.1979)
  line L152 (-60.7954, 78.1979) -> (-60.7954, 78.5832)
  line L153 (-60.7954, 78.5832) -> (-59.6444, 78.5832)
  spline S166 degree 2 poles (-59.6444, 78.5832) (-59.8, 78.7561) (-59.963, 79.0896) (-59.963, 79.2773) knots 0 0 0 1 2 2 2
  spline S167 degree 2 poles (-59.963, 79.2773) (-59.963, 79.6132) (-59.5184, 79.9936) (-59.096, 79.9936) knots 0 0 0 1 2 2 2
  line L154 (-59.096, 79.9936) -> (-57.6115, 79.9936)
  spline S168 degree 2 poles (-57.5597, 81.5275) (-57.5597, 80.9792) (-58.1747, 80.3765) (-58.7428, 80.3765) knots 0 0 0 1 2 2 2
  spline S169 degree 2 poles (-58.7428, 80.3765) (-59.301, 80.3765) (-59.963, 80.9619) (-59.963, 81.4336) knots 0 0 0 1 2 2 2
  spline S170 degree 2 poles (-59.963, 81.4336) (-59.963, 81.6461) (-59.8395, 81.9746) (-59.7086, 82.0956) knots 0 0 0 1 2 2 2
  spline S171 degree 2 poles (-59.7086, 82.0956) (-59.5777, 82.2191) (-59.1997, 82.35) (-58.9256, 82.35) knots 0 0 0 1 2 2 2
  line L155 (-58.9256, 82.35) -> (-58.7156, 82.35)
  line L156 (-58.7156, 82.35) -> (-58.7156, 80.7667)
  spline S172 degree 2 poles (-58.7156, 80.7667) (-58.318, 80.7667) (-57.8956, 81.1669) (-57.8956, 81.5226) knots 0 0 0 1 2 2 2
  spline S173 degree 2 poles (-57.8956, 81.5226) (-57.8956, 81.6485) (-57.9524, 81.8931) (-57.9969, 81.9919) knots 0 0 0 1 2 2 2
  spline S174 degree 2 poles (-57.9969, 81.9919) (-58.0463, 82.0956) (-58.1327, 82.2389) (-58.1722, 82.2858) knots 0 0 0 1 2 2 2
  line L157 (-58.1722, 82.2858) -> (-58.1722, 82.308)
  line L158 (-58.1722, 82.308) -> (-57.7523, 82.308)
  spline S175 degree 2 poles (-57.7523, 82.308) (-57.7251, 82.2413) (-57.6461, 82.0388) (-57.6239, 81.9597) knots 0 0 0 1 2 2 2
  spline S176 degree 2 poles (-57.6239, 81.9597) (-57.5918, 81.8486) (-57.5597, 81.6658) (-57.5597, 81.5275) knots 0 0 0 1 2 2 2
  spline S177 degree 2 poles (-59.0096, 81.9746) (-59.1652, 81.9696) (-59.3924, 81.9054) (-59.469, 81.8437) knots 0 0 0 1 2 2 2
  spline S178 degree 2 poles (-59.469, 81.8437) (-59.5554, 81.777) (-59.6468, 81.567) (-59.6468, 81.4114) knots 0 0 0 1 2 2 2
  spline S179 degree 2 poles (-59.6468, 81.4114) (-59.6468, 81.2583) (-59.5554, 81.0434) (-59.4665, 80.9545) knots 0 0 0 1 2 2 2
  spline S180 degree 2 poles (-59.4665, 80.9545) (-59.3751, 80.868) (-59.1553, 80.7791) (-59.0096, 80.7667) knots 0 0 0 1 2 2 2
  line L159 (-59.0096, 80.7667) -> (-59.0096, 81.9746)
  line L160 (-60.4249, 85.2523) -> (-60.4249, 85.2325)
  spline S181 degree 2 poles (-60.4249, 85.2325) (-60.4446, 85.1806) (-60.4792, 84.988) (-60.4792, 84.9114) knots 0 0 0 1 2 2 2
  spline S182 degree 2 poles (-60.4792, 84.9114) (-60.4792, 84.6694) (-60.2619, 84.4619) (-59.9753, 84.4619) knots 0 0 0 1 2 2 2
  line L161 (-59.9753, 84.4619) -> (-59.8988, 84.4619)
  line L162 (-59.8988, 84.4619) -> (-59.8988, 85.0991)
  line L163 (-59.8988, 85.0991) -> (-59.5801, 85.0991)
  line L164 (-59.5801, 85.0991) -> (-59.5801, 84.4742)
  line L165 (-59.5801, 84.4742) -> (-57.6115, 84.4742)
  line L166 (-57.6115, 84.4742) -> (-57.6115, 84.0889)
  line L167 (-57.6115, 84.0889) -> (-59.5801, 84.0889)
  line L168 (-59.5801, 84.0889) -> (-59.5801, 83.8296)
  line L169 (-59.5801, 83.8296) -> (-59.8988, 83.8296)
  line L170 (-59.8988, 83.8296) -> (-59.8988, 84.0889)
  line L171 (-59.8988, 84.0889) -> (-59.9753, 84.0889)
  spline S183 degree 2 poles (-59.9753, 84.0889) (-60.3854, 84.0889) (-60.8151, 84.4866) (-60.8151, 84.8571) knots 0 0 0 1 2 2 2
  spline S184 degree 2 poles (-60.8151, 84.8571) (-60.8151, 84.9633) (-60.7929, 85.1683) (-60.7781, 85.2523) knots 0 0 0 1 2 2 2
  line L172 (-60.7781, 85.2523) -> (-60.4249, 85.2523)
  line L173 (-57.6115, 87.1616) -> (-57.6115, 86.7763)
  line L174 (-57.6115, 86.7763) -> (-57.8635, 86.7763)
  spline S185 degree 2 poles (-57.8635, 86.7763) (-57.7079, 86.5984) (-57.5473, 86.2798) (-57.5473, 86.0822) knots 0 0 0 1 2 2 2
  spline S186 degree 2 poles (-57.5473, 86.0822) (-57.5473, 85.934) (-57.6461, 85.6697) (-57.7523, 85.5734) knots 0 0 0 1 2 2 2
  spline S187 degree 2 poles (-57.7523, 85.5734) (-57.8585, 85.4746) (-58.1821, 85.3659) (-58.4143, 85.3659) knots 0 0 0 1 2 2 2
  line L175 (-58.4143, 85.3659) -> (-59.8988, 85.3659)
  line L176 (-59.8988, 85.3659) -> (-59.8988, 85.7512)
  line L177 (-59.8988, 85.7512) -> (-58.5946, 85.7512)
  spline S188 degree 2 poles (-58.5946, 85.7512) (-58.4118, 85.7512) (-58.1722, 85.7784) (-58.0833, 85.8253) knots 0 0 0 1 2 2 2
  spline S189 degree 2 poles (-58.0833, 85.8253) (-57.9944, 85.8723) (-57.9129, 86.0328) (-57.9129, 86.1835) knots 0 0 0 1 2 2 2
  spline S190 degree 2 poles (-57.9129, 86.1835) (-57.9129, 86.3243) (-58.0734, 86.6429) (-58.1895, 86.7763) knots 0 0 0 1 2 2 2
  line L178 (-58.1895, 86.7763) -> (-59.8988, 86.7763)
  line L179 (-59.8988, 86.7763) -> (-59.8988, 87.1616)
  line L180 (-59.8988, 87.1616) -> (-57.6115, 87.1616)
  line L181 (-57.6115, 89.5155) -> (-57.6115, 89.1302)
  line L182 (-57.6115, 89.1302) -> (-58.9157, 89.1302)
  spline S191 degree 2 poles (-58.9157, 89.1302) (-59.0738, 89.1302) (-59.3455, 89.1006) (-59.427, 89.0561) knots 0 0 0 1 2 2 2
  spline S192 degree 2 poles (-59.427, 89.0561) (-59.5134, 89.0092) (-59.5974, 88.8412) (-59.5974, 88.698) knots 0 0 0 1 2 2 2
  spline S193 degree 2 poles (-59.5974, 88.698) (-59.5974, 88.5547) (-59.4443, 88.2509) (-59.3208, 88.1051) knots 0 0 0 1 2 2 2
  line L183 (-59.3208, 88.1051) -> (-57.6115, 88.1051)
  line L184 (-57.6115, 88.1051) -> (-57.6115, 87.7198)
  line L185 (-57.6115, 87.7198) -> (-59.8988, 87.7198)
  line L186 (-59.8988, 87.7198) -> (-59.8988, 88.1051)
  line L187 (-59.8988, 88.1051) -> (-59.6444, 88.1051)
  spline S194 degree 2 poles (-59.6444, 88.1051) (-59.8, 88.278) (-59.963, 88.6115) (-59.963, 88.7992) knots 0 0 0 1 2 2 2
  spline S195 degree 2 poles (-59.963, 88.7992) (-59.963, 89.1351) (-59.5184, 89.5155) (-59.096, 89.5155) knots 0 0 0 1 2 2 2
  line L188 (-59.096, 89.5155) -> (-57.6115, 89.5155)
  line L189 (-57.6115, 91.8522) -> (-57.6115, 91.4668)
  line L190 (-57.6115, 91.4668) -> (-58.9157, 91.4668)
  spline S196 degree 2 poles (-58.9157, 91.4668) (-59.0738, 91.4668) (-59.3455, 91.4372) (-59.427, 91.3927) knots 0 0 0 1 2 2 2
  spline S197 degree 2 poles (-59.427, 91.3927) (-59.5134, 91.3458) (-59.5974, 91.1778) (-59.5974, 91.0346) knots 0 0 0 1 2 2 2
  spline S198 degree 2 poles (-59.5974, 91.0346) (-59.5974, 90.8913) (-59.4443, 90.5875) (-59.3208, 90.4418) knots 0 0 0 1 2 2 2
  line L191 (-59.3208, 90.4418) -> (-57.6115, 90.4418)
  line L192 (-57.6115, 90.4418) -> (-57.6115, 90.0565)
  line L193 (-57.6115, 90.0565) -> (-59.8988, 90.0565)
  line L194 (-59.8988, 90.0565) -> (-59.8988, 90.4418)
  line L195 (-59.8988, 90.4418) -> (-59.6444, 90.4418)
  spline S199 degree 2 poles (-59.6444, 90.4418) (-59.8, 90.6147) (-59.963, 90.9481) (-59.963, 91.1359) knots 0 0 0 1 2 2 2
  spline S200 degree 2 poles (-59.963, 91.1359) (-59.963, 91.4718) (-59.5184, 91.8522) (-59.096, 91.8522) knots 0 0 0 1 2 2 2
  line L196 (-59.096, 91.8522) -> (-57.6115, 91.8522)
  line L197 (-59.8988, 94.1888) -> (-56.7693, 92.9587)
  line L198 (-56.7693, 92.9587) -> (-56.7693, 92.5462)
  line L199 (-56.7693, 92.5462) -> (-57.7227, 92.9563)
  line L200 (-57.7227, 92.9563) -> (-59.8988, 92.1263)
  line L201 (-59.8988, 92.1263) -> (-59.8988, 92.5413)
  line L202 (-59.8988, 92.5413) -> (-58.2043, 93.1662)
  line L203 (-58.2043, 93.1662) -> (-59.8988, 93.7887)
  line L204 (-59.8988, 93.7887) -> (-59.8988, 94.1888)
  spline S201 degree 2 poles (-58.7551, 97.6691) (-58.1772, 97.6691) (-57.5473, 97.1133) (-57.5473, 96.6489) knots 0 0 0 1 2 2 2
  spline S202 degree 2 poles (-57.5473, 96.6489) (-57.5473, 96.1722) (-58.1969, 95.6263) (-58.7551, 95.6263) knots 0 0 0 1 2 2 2
  spline S203 degree 2 poles (-58.7551, 95.6263) (-59.3282, 95.6263) (-59.963, 96.1895) (-59.963, 96.6489) knots 0 0 0 1 2 2 2
  spline S204 degree 2 poles (-59.963, 96.6489) (-59.963, 97.1133) (-59.3307, 97.6691) (-58.7551, 97.6691) knots 0 0 0 1 2 2 2
  spline S205 degree 2 poles (-58.7551, 97.2714) (-59.1997, 97.2714) (-59.632, 96.9478) (-59.632, 96.6489) knots 0 0 0 1 2 2 2
  spline S206 degree 2 poles (-59.632, 96.6489) (-59.632, 96.3501) (-59.1997, 96.024) (-58.7551, 96.024) knots 0 0 0 1 2 2 2
  spline S207 degree 2 poles (-58.7551, 96.024) (-58.3229, 96.024) (-57.8783, 96.3501) (-57.8783, 96.6489) knots 0 0 0 1 2 2 2
  spline S208 degree 2 poles (-57.8783, 96.6489) (-57.8783, 96.9453) (-58.3155, 97.2714) (-58.7551, 97.2714) knots 0 0 0 1 2 2 2
  line L205 (-57.6115, 98.457) -> (-57.6115, 98.0717)
  line L206 (-57.6115, 98.0717) -> (-60.7954, 98.0717)
  line L207 (-60.7954, 98.0717) -> (-60.7954, 98.457)
  line L208 (-60.7954, 98.457) -> (-57.6115, 98.457)
  spline S209 degree 2 poles (-57.5597, 100.0156) (-57.5597, 99.4672) (-58.1747, 98.8645) (-58.7428, 98.8645) knots 0 0 0 1 2 2 2
  spline S210 degree 2 poles (-58.7428, 98.8645) (-59.301, 98.8645) (-59.963, 99.4499) (-59.963, 99.9217) knots 0 0 0 1 2 2 2
  spline S211 degree 2 poles (-59.963, 99.9217) (-59.963, 100.1341) (-59.8395, 100.4626) (-59.7086, 100.5837) knots 0 0 0 1 2 2 2
  spline S212 degree 2 poles (-59.7086, 100.5837) (-59.5777, 100.7072) (-59.1997, 100.8381) (-58.9256, 100.8381) knots 0 0 0 1 2 2 2
  line L209 (-58.9256, 100.8381) -> (-58.7156, 100.8381)
  line L210 (-58.7156, 100.8381) -> (-58.7156, 99.2548)
  spline S213 degree 2 poles (-58.7156, 99.2548) (-58.318, 99.2548) (-57.8956, 99.6549) (-57.8956, 100.0106) knots 0 0 0 1 2 2 2
  spline S214 degree 2 poles (-57.8956, 100.0106) (-57.8956, 100.1366) (-57.9524, 100.3811) (-57.9969, 100.4799) knots 0 0 0 1 2 2 2
  spline S215 degree 2 poles (-57.9969, 100.4799) (-58.0463, 100.5837) (-58.1327, 100.7269) (-58.1722, 100.7739) knots 0 0 0 1 2 2 2
  line L211 (-58.1722, 100.7739) -> (-58.1722, 100.7961)
  line L212 (-58.1722, 100.7961) -> (-57.7523, 100.7961)
  spline S216 degree 2 poles (-57.7523, 100.7961) (-57.7251, 100.7294) (-57.6461, 100.5269) (-57.6239, 100.4478) knots 0 0 0 1 2 2 2
  spline S217 degree 2 poles (-57.6239, 100.4478) (-57.5918, 100.3367) (-57.5597, 100.1539) (-57.5597, 100.0156) knots 0 0 0 1 2 2 2
  spline S218 degree 2 poles (-59.0096, 100.4626) (-59.1652, 100.4577) (-59.3924, 100.3935) (-59.469, 100.3317) knots 0 0 0 1 2 2 2
  spline S219 degree 2 poles (-59.469, 100.3317) (-59.5554, 100.265) (-59.6468, 100.0551) (-59.6468, 99.8995) knots 0 0 0 1 2 2 2
  spline S220 degree 2 poles (-59.6468, 99.8995) (-59.6468, 99.7463) (-59.5554, 99.5314) (-59.4665, 99.4425) knots 0 0 0 1 2 2 2
  spline S221 degree 2 poles (-59.4665, 99.4425) (-59.3751, 99.3561) (-59.1553, 99.2672) (-59.0096, 99.2548) knots 0 0 0 1 2 2 2
  line L213 (-59.0096, 99.2548) -> (-59.0096, 100.4626)
  line L214 (-57.6115, 102.987) -> (-57.6115, 102.6017)
  line L215 (-57.6115, 102.6017) -> (-57.8437, 102.6017)
  spline S222 degree 2 poles (-57.8437, 102.6017) (-57.7696, 102.5128) (-57.6708, 102.3818) (-57.6288, 102.2929) knots 0 0 0 1 2 2 2
  spline S223 degree 2 poles (-57.6288, 102.2929) (-57.5893, 102.2114) (-57.5473, 102.036) (-57.5473, 101.9199) knots 0 0 0 1 2 2 2
  spline S224 degree 2 poles (-57.5473, 101.9199) (-57.5473, 101.7322) (-57.7029, 101.4161) (-57.8536, 101.3049) knots 0 0 0 1 2 2 2
  spline S225 degree 2 poles (-57.8536, 101.3049) (-58.0043, 101.1938) (-58.4489, 101.0703) (-58.7379, 101.0703) knots 0 0 0 1 2 2 2
  spline S226 degree 2 poles (-58.7379, 101.0703) (-59.0392, 101.0703) (-59.4789, 101.2259) (-59.6444, 101.3617) knots 0 0 0 1 2 2 2
  spline S227 degree 2 poles (-59.6444, 101.3617) (-59.7926, 101.4877) (-59.963, 101.8409) (-59.963, 102.036) knots 0 0 0 1 2 2 2
  spline S228 degree 2 poles (-59.963, 102.036) (-59.963, 102.2065) (-59.8864, 102.4609) (-59.8074, 102.6017) knots 0 0 0 1 2 2 2
  line L216 (-59.8074, 102.6017) -> (-60.7954, 102.6017)
  line L217 (-60.7954, 102.6017) -> (-60.7954, 102.987)
  line L218 (-60.7954, 102.987) -> (-57.6115, 102.987)
  line L219 (-58.1673, 102.6017) -> (-59.4887, 102.6017)
  spline S229 degree 2 poles (-59.4887, 102.6017) (-59.5579, 102.4584) (-59.6098, 102.2312) (-59.6098, 102.1003) knots 0 0 0 1 2 2 2
  spline S230 degree 2 poles (-59.6098, 102.1003) (-59.6098, 101.8039) (-59.1652, 101.4679) (-58.7453, 101.4679) knots 0 0 0 1 2 2 2
  spline S231 degree 2 poles (-58.7453, 101.4679) (-58.3402, 101.4679) (-57.9129, 101.7248) (-57.9129, 102.0089) knots 0 0 0 1 2 2 2
  spline S232 degree 2 poles (-57.9129, 102.0089) (-57.9129, 102.1595) (-58.0512, 102.4658) (-58.1673, 102.6017) knots 0 0 0 1 2 2 2
  line L220 (-57.6115, 106.65) -> (-57.6115, 106.2647)
  line L221 (-57.6115, 106.2647) -> (-58.9157, 106.2647)
  spline S233 degree 2 poles (-58.9157, 106.2647) (-59.0738, 106.2647) (-59.3455, 106.2351) (-59.427, 106.1906) knots 0 0 0 1 2 2 2
  spline S234 degree 2 poles (-59.427, 106.1906) (-59.5134, 106.1437) (-59.5974, 105.9757) (-59.5974, 105.8325) knots 0 0 0 1 2 2 2
  spline S235 degree 2 poles (-59.5974, 105.8325) (-59.5974, 105.6892) (-59.4443, 105.3854) (-59.3208, 105.2397) knots 0 0 0 1 2 2 2
  line L222 (-59.3208, 105.2397) -> (-57.6115, 105.2397)
  line L223 (-57.6115, 105.2397) -> (-57.6115, 104.8543)
  line L224 (-57.6115, 104.8543) -> (-60.7954, 104.8543)
  line L225 (-60.7954, 104.8543) -> (-60.7954, 105.2397)
  line L226 (-60.7954, 105.2397) -> (-59.6444, 105.2397)
  spline S236 degree 2 poles (-59.6444, 105.2397) (-59.8, 105.4126) (-59.963, 105.746) (-59.963, 105.9337) knots 0 0 0 1 2 2 2
  spline S237 degree 2 poles (-59.963, 105.9337) (-59.963, 106.2696) (-59.5184, 106.65) (-59.096, 106.65) knots 0 0 0 1 2 2 2
  line L227 (-59.096, 106.65) -> (-57.6115, 106.65)
  spline S238 degree 2 poles (-57.5597, 108.1839) (-57.5597, 107.6356) (-58.1747, 107.0329) (-58.7428, 107.0329) knots 0 0 0 1 2 2 2
  spline S239 degree 2 poles (-58.7428, 107.0329) (-59.301, 107.0329) (-59.963, 107.6183) (-59.963, 108.09) knots 0 0 0 1 2 2 2
  spline S240 degree 2 poles (-59.963, 108.09) (-59.963, 108.3025) (-59.8395, 108.631) (-59.7086, 108.752) knots 0 0 0 1 2 2 2
  spline S241 degree 2 poles (-59.7086, 108.752) (-59.5777, 108.8755) (-59.1997, 109.0064) (-58.9256, 109.0064) knots 0 0 0 1 2 2 2
  line L228 (-58.9256, 109.0064) -> (-58.7156, 109.0064)
  line L229 (-58.7156, 109.0064) -> (-58.7156, 107.4231)
  spline S242 degree 2 poles (-58.7156, 107.4231) (-58.318, 107.4231) (-57.8956, 107.8233) (-57.8956, 108.179) knots 0 0 0 1 2 2 2
  spline S243 degree 2 poles (-57.8956, 108.179) (-57.8956, 108.3049) (-57.9524, 108.5495) (-57.9969, 108.6483) knots 0 0 0 1 2 2 2
  spline S244 degree 2 poles (-57.9969, 108.6483) (-58.0463, 108.752) (-58.1327, 108.8953) (-58.1722, 108.9422) knots 0 0 0 1 2 2 2
  line L230 (-58.1722, 108.9422) -> (-58.1722, 108.9644)
  line L231 (-58.1722, 108.9644) -> (-57.7523, 108.9644)
  spline S245 degree 2 poles (-57.7523, 108.9644) (-57.7251, 108.8977) (-57.6461, 108.6952) (-57.6239, 108.6162) knots 0 0 0 1 2 2 2
  spline S246 degree 2 poles (-57.6239, 108.6162) (-57.5918, 108.505) (-57.5597, 108.3222) (-57.5597, 108.1839) knots 0 0 0 1 2 2 2
  spline S247 degree 2 poles (-59.0096, 108.631) (-59.1652, 108.626) (-59.3924, 108.5618) (-59.469, 108.5001) knots 0 0 0 1 2 2 2
  spline S248 degree 2 poles (-59.469, 108.5001) (-59.5554, 108.4334) (-59.6468, 108.2234) (-59.6468, 108.0678) knots 0 0 0 1 2 2 2
  spline S249 degree 2 poles (-59.6468, 108.0678) (-59.6468, 107.9147) (-59.5554, 107.6998) (-59.4665, 107.6109) knots 0 0 0 1 2 2 2
  spline S250 degree 2 poles (-59.4665, 107.6109) (-59.3751, 107.5244) (-59.1553, 107.4355) (-59.0096, 107.4231) knots 0 0 0 1 2 2 2
  line L232 (-59.0096, 107.4231) -> (-59.0096, 108.631)
  line L233 (-59.4863, 110.6095) -> (-59.4863, 110.5897)
  spline S251 degree 2 poles (-59.4863, 110.5897) (-59.4986, 110.5452) (-59.5036, 110.4489) (-59.5036, 110.3822) knots 0 0 0 1 2 2 2
  spline S252 degree 2 poles (-59.5036, 110.3822) (-59.5036, 110.2266) (-59.3677, 109.9203) (-59.2343, 109.782) knots 0 0 0 1 2 2 2
  line L234 (-59.2343, 109.782) -> (-57.6115, 109.782)
  line L235 (-57.6115, 109.782) -> (-57.6115, 109.3967)
  line L236 (-57.6115, 109.3967) -> (-59.8988, 109.3967)
  line L237 (-59.8988, 109.3967) -> (-59.8988, 109.782)
  line L238 (-59.8988, 109.782) -> (-59.5579, 109.782)
  spline S253 degree 2 poles (-59.5579, 109.782) (-59.7456, 109.992) (-59.8988, 110.3057) (-59.8988, 110.4539) knots 0 0 0 1 2 2 2
  spline S254 degree 2 poles (-59.8988, 110.4539) (-59.8988, 110.5131) (-59.8938, 110.5724) (-59.8864, 110.6095) knots 0 0 0 1 2 2 2
  line L239 (-59.8864, 110.6095) -> (-59.4863, 110.6095)
  spline S255 degree 2 poles (-57.5597, 111.9013) (-57.5597, 111.3529) (-58.1747, 110.7503) (-58.7428, 110.7503) knots 0 0 0 1 2 2 2
  spline S256 degree 2 poles (-58.7428, 110.7503) (-59.301, 110.7503) (-59.963, 111.3357) (-59.963, 111.8074) knots 0 0 0 1 2 2 2
  spline S257 degree 2 poles (-59.963, 111.8074) (-59.963, 112.0198) (-59.8395, 112.3484) (-59.7086, 112.4694) knots 0 0 0 1 2 2 2